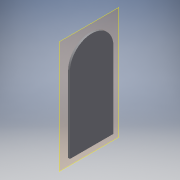
# Autodesk Inventor part: pOOPOODOOR
Saved by Autodesk Inventor 2019 (Build 230136000, 136)
## iProperties
Created: 2019-11-13
Part Number: pOOPOODOOR
Material: Generic
Document SubType Name: Modeling
Designer: Administrator
Density: 1 g/cm^3
Appearance: Default
Author: Administrator
Autodesk Inventor part; units mm, degrees
ref_plane "YZ Plane" through (0, 0, 0) normal (1, 0, 0) x (0, 1, 0)
ref_plane "XZ Plane" through (0, 0, 0) normal (0, 1, 0) x (-1, 0, 0)
ref_plane "XY Plane" through (0, 0, 0) normal (0, 0, 1) x (1, 0, 0)
ref_plane "Work Plane1" through (2731.4011, -1060.2356, 2291.4203) normal (1, 0, 0) x (0, 1, 0)
sketch "Sketch1" plane through (2731.4011, -1060.2356, 2291.4203) normal (1, 0, 0) x (0, 1, 0)
  line L0 (79.0938, -145.4532) -> (1857.0938, -145.4532)
  line L1 (1857.0938, -1161.4532) -> (79.0938, -1161.4532)
  line L2 (79.0938, -1161.4532) -> (79.0938, -145.4532)
  arc A0 (1857.0938, -1161.4532) -> (1857.0938, -145.4532) centre (1857.0938, -653.4532) ccw
  point P0 (1060.2356, -2291.4203)
  constraints: 6 end point, 2 point on circle, 2 tangent, 1 centre point, 1 horizontal, 1 parallel
extrude "Extrusion1" add sketch "Sketch1" along normal blind 42.926
body "Solid1"
